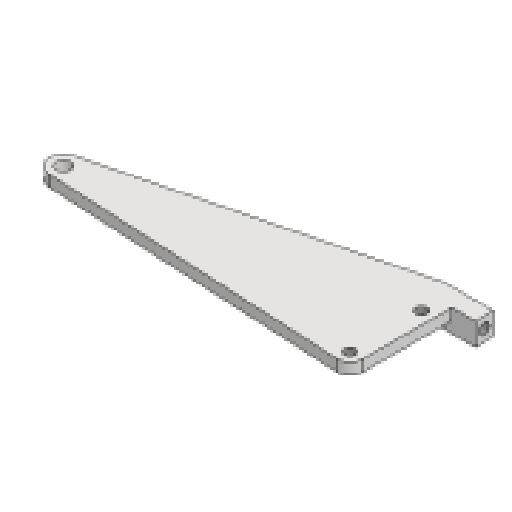
# Autodesk Inventor part: intakeSlidesWheelHolder
Saved by Autodesk Inventor 2023 (Build 270158000, 158)
## iProperties
Created: 2022-11-03
Part Number: intakeSlidesWheelHolder
Material: Generic
Document SubType Name: Modeling
Designer: deli
Density: 1 g/cm^3
Appearance: Default
Author: deli
Autodesk Inventor part; units mm, degrees
ref_plane "YZ Plane" through (0, 0, 0) normal (1, 0, 0) x (0, 1, 0)
ref_plane "XZ Plane" through (0, 0, 0) normal (0, 1, 0) x (-1, 0, 0)
ref_plane "XY Plane" through (0, 0, 0) normal (0, 0, 1) x (1, 0, 0)
sketch "Sketch1" plane through (0, 0, 0) normal (0, 1, 0) x (-1, 0, 0)
  circle A0 centre (28.9139, 46.0513) radius 1.5
  circle A1 centre (28.9139, 26.0513) radius 1.5
  arc A2 (32.4139, 46.0513) -> (25.4139, 46.0513) centre (28.9139, 46.0513) ccw
  line L0 (32.4139, 46.0513) -> (32.4139, 16.0513)
  line L1 (32.4139, 16.0513) -> (18.9139, 16.0513)
  line L2 (25.4139, 21.0513) -> (25.4139, 46.0513)
  line L3 (18.9139, 16.0513) -> (18.9139, 21.0513)
  line L4 (18.9139, 21.0513) -> (25.4139, 21.0513)
  line L5 (32.4139, 16.0513) -> (118.863, 37.1655)
  arc A3 (118.863, 37.1655) -> (118.1159, 45.0462) centre (117.9139, 41.0513) ccw
  line L6 (118.1159, 45.0462) -> (29.0906, 49.5468)
  circle A4 centre (117.9139, 41.0513) radius 2
  point P0 (0, 0)
  dimension "d0" = 3
  dimension "d1" = 2
  dimension "d2" = 20
  dimension "d3" = 10
  dimension "d20" = 10
  dimension "d27" = 8
  dimension "d28" = 4
  dimension "d29" = 85.5
  dimension "d30" = 3.5
  dimension "d32" = 5
  constraints: 14 end point, 5 centre point, 5 point on circle, 5 tangent, 2 coincident, 1 equal radius, 1 parallel, 1 perpendicular, 1 vertical
  measures "d0" diameter of A0
  measures "d1" radial gap between concentric circles of A2 A0
  measures "d2" distance of A0.centre A1.centre
  measures "d3" distance from line of L1 A1.centre
  measures "d20" distance from line of A1.centre L3
  measures "d27" diameter of A3
  measures "d28" diameter of A4
  measures "d29" distance from line of L0 A4.centre
  measures "d30" distance from line of A1.centre L0
  measures "d32" distance of L1.end L3.end
extrude "Extrusion1" add sketch "Sketch1" along normal blind 3.175
sketch "Sketch2" plane through (0, 3.175, 0) normal (0, 1, 0) x (1, 0, 0)
  line L0 (-32.4139, -16.0513) -> (-18.9139, -16.0513)
  line L1 (-18.9139, -16.0513) -> (-18.9139, -21.0513)
  line L2 (-18.9139, -21.0513) -> (-32.4139, -21.0513)
  line L3 (-32.4139, -21.0513) -> (-32.4139, -16.0513)
  point P0 (0, 0)
  constraints: 8 end point, 2 coincident, 2 parallel, 1 horizontal, 1 perpendicular
extrude "Extrusion2" add sketch "Sketch2" against normal blind 6.35
thread "Thread1" size "M3x0.5" class "6H" standard "ANSI Metric M Profile" full length
thread "Thread3" size "M3x0.5" class "6H" standard "ANSI Metric M Profile" full length
sketch "Sketch4" plane through (-18.9139, 0, 21.0513) normal (1, 0, 0) x (0, 0, 1)
  line L0 (0, 0) -> (25, 0) projected
  circle A0 centre (-2.5, 0) radius 1.5
  line L1 (0, 0) -> (0, 3.175) construction
  line L2 (-5, -3.175) -> (25, -3.175) construction
  line L3 (0, 3.175) -> (-5, -3.175) construction
  point P0 (-21.0513, 0)
  dimension "d26" = 3
  constraints: 2 end point, 1 centre point, 1 coincident, 1 midpoint
  measures "d26" diameter of A0
extrude "Extrusion4" cut sketch "Sketch4" against normal blind 8
thread "Thread4" size "M3x0.5" class "6H" standard "ANSI Metric M Profile" full length
body "Solid1"
